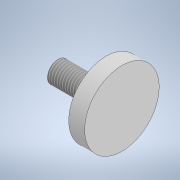
# Autodesk Inventor part: Knob
Saved by Autodesk Inventor 2022 (Build 260153000, 153)
## iProperties
Created: 2021-06-24
Part Number: Knob
Material: Generic
Document SubType Name: Modeling
Designer: Admin
Density: 1 g/cm^3
Appearance: Default
Author: Admin
Autodesk Inventor part; units mm, degrees
ref_plane "YZ Plane" through (0, 0, 0) normal (1, 0, 0) x (0, 1, 0)
ref_plane "XZ Plane" through (0, 0, 0) normal (0, 1, 0) x (-1, 0, 0)
ref_plane "XY Plane" through (0, 0, 0) normal (0, 0, 1) x (1, 0, 0)
sketch "Sketch1" plane through (0, 0, 0) normal (0, 0, 1) x (1, 0, 0)
  line L0 (0, 0) -> (0, 10)
  line L1 (0, 10) -> (35, 10)
  line L2 (35, 10) -> (35, 15)
  line L3 (35, 15) -> (45, 15)
  line L4 (45, 15) -> (45, 35)
  line L5 (45, 35) -> (60, 35)
  line L6 (60, 35) -> (60, 0)
  line L7 (60, 0) -> (0, 0)
  dimension "d4" = 10
  dimension "d5" = 35
  dimension "d6" = 5
  dimension "d7" = 10
  dimension "d8" = 20
  dimension "d9" = 15
  constraints: 16 end point, 5 perpendicular, 2 horizontal, 1 vertical
  measures "d4" distance of L0.start L0.end
  measures "d5" distance of L0.end L1.end
  measures "d6" distance of L1.end L2.end
  measures "d7" distance of L2.end L3.end
  measures "d8" distance of L3.end L4.end
  measures "d9" distance of L4.end L5.end
revolve "Revolution1" add sketch "Sketch1" angle 360 about axis through (60, 0, 0) along (-1, 0, 0)
thread "Thread1" size "M20x2.5" class "6g" standard "ANSI Metric M Profile" full length
body "Solid1"
